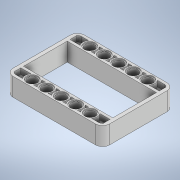
# Autodesk Inventor part: magazine-adapter
Saved by Autodesk Inventor 2021 (Build 250183000, 183)
## iProperties
Created: 2024-03-14
Part Number: magazine-adapter
Material: Generic
Document SubType Name: Modeling
Designer: 22hamfri
Density: 1 g/cm^3
Appearance: Default
Author: 22hamfri
Autodesk Inventor part; units mm, degrees
ref_plane "YZ Plane" through (0, 0, 0) normal (1, 0, 0) x (0, 1, 0)
ref_plane "XZ Plane" through (0, 0, 0) normal (0, 1, 0) x (-1, 0, 0)
ref_plane "XY Plane" through (0, 0, 0) normal (0, 0, 1) x (1, 0, 0)
sketch "Sketch1" plane through (0, 0, 0) normal (0, 1, 0) x (-1, 0, 0)
  line L0 (-24.5, 12) -> (24.5, 12)
  line L1 (24.5, 12) -> (24.5, -12)
  line L2 (24.5, -12) -> (-24.5, -12)
  line L3 (-24.5, -12) -> (-24.5, 12)
  line L4 (-24.5, 12) -> (24.5, -12) construction
  line L5 (24.5, 12) -> (-24.5, -12) construction
  line L6 (-26.5, 19.6) -> (26.5, 19.6)
  line L7 (26.5, 19.6) -> (26.5, -19.6)
  line L8 (26.5, -19.6) -> (-26.5, -19.6)
  line L9 (-26.5, -19.6) -> (-26.5, 19.6)
  line L10 (-26.5, 19.6) -> (26.5, -19.6) construction
  line L11 (26.5, 19.6) -> (-26.5, -19.6) construction
  circle A0 centre (0, -15.8) radius 2.575
  circle A1 centre (0, -15.8) radius 3.1
  circle A2 centre (0, -15.8) radius 3.8
  circle A3 centre (-7.97, -15.8) radius 2.575
  circle A4 centre (-7.97, -15.8) radius 3.1
  circle A5 centre (-7.97, -15.8) radius 3.8
  circle A6 centre (-15.94, -15.8) radius 2.575
  circle A7 centre (-15.94, -15.8) radius 3.1
  circle A8 centre (-15.94, -15.8) radius 3.8
  circle A9 centre (7.97, -15.8) radius 2.575
  circle A10 centre (7.97, -15.8) radius 3.1
  circle A11 centre (7.97, -15.8) radius 3.8
  circle A12 centre (0, -15.8) radius 2.575
  circle A13 centre (0, -15.8) radius 3.1
  circle A14 centre (0, -15.8) radius 3.8
  circle A15 centre (-7.97, -15.8) radius 2.575
  circle A16 centre (-7.97, -15.8) radius 3.1
  circle A17 centre (-7.97, -15.8) radius 3.8
  circle A18 centre (15.94, -15.8) radius 2.575
  circle A19 centre (15.94, -15.8) radius 3.1
  circle A20 centre (15.94, -15.8) radius 3.8
  circle A21 centre (7.97, -15.8) radius 2.575
  circle A22 centre (7.97, -15.8) radius 3.1
  circle A23 centre (7.97, -15.8) radius 3.8
  circle A24 centre (0, -15.8) radius 2.575
  circle A25 centre (0, -15.8) radius 3.1
  circle A26 centre (0, -15.8) radius 3.8
  line L12 (0, 0) -> (0, -19.6)
  line L13 (18.9649, -13.5) -> (24.5, -13.5)
  line L14 (24.5, -13.5) -> (24.5, -17.2318)
  line L15 (12.9151, -13.5) -> (10.9949, -13.5)
  line L16 (12.9151, -18.1) -> (10.9949, -18.1)
  line L17 (4.9451, -13.5) -> (3.0249, -13.5)
  line L18 (4.9451, -18.1) -> (3.0249, -18.1)
  line L19 (-3.0249, -13.5) -> (-4.9451, -13.5)
  line L20 (-3.0249, -18.1) -> (-4.9451, -18.1)
  line L21 (-10.9949, -13.5) -> (-12.9151, -13.5)
  line L22 (-10.9949, -18.1) -> (-12.9151, -18.1)
  line L23 (-18.9649, -13.5) -> (-24.5, -13.5)
  line L24 (-24.5, -13.5) -> (-24.5, -17.2318)
  arc A27 (22.7, -19.6) -> (26.5, -15.8) centre (22.7, -15.8) ccw
  arc A28 (22.7, -18.1) -> (24.5, -17.2318) centre (22.7, -15.8) ccw
  line L25 (22.7, -18.1) -> (18.9649, -18.1)
  arc A29 (-26.5, -15.8) -> (-22.7, -19.6) centre (-22.7, -15.8) ccw
  arc A30 (-24.5, -17.2318) -> (-22.7, -18.1) centre (-22.7, -15.8) ccw
  line L26 (-22.7, -18.1) -> (-18.9649, -18.1)
  line L27 (26.5, 0) -> (-26.5, 0)
  line L28 (24.5, 12) -> (-24.5, 12)
  line L29 (26.5, 19.6) -> (-26.5, 19.6)
  circle A31 centre (0, 15.8) radius 2.575
  circle A32 centre (0, 15.8) radius 3.1
  circle A33 centre (0, 15.8) radius 3.8
  circle A34 centre (-7.97, 15.8) radius 2.575
  circle A35 centre (-7.97, 15.8) radius 3.1
  circle A36 centre (-7.97, 15.8) radius 3.8
  circle A37 centre (-15.94, 15.8) radius 2.575
  circle A38 centre (-15.94, 15.8) radius 3.1
  circle A39 centre (-15.94, 15.8) radius 3.8
  circle A40 centre (7.97, 15.8) radius 2.575
  circle A41 centre (7.97, 15.8) radius 3.1
  circle A42 centre (7.97, 15.8) radius 3.8
  circle A43 centre (0, 15.8) radius 2.575
  circle A44 centre (0, 15.8) radius 3.1
  circle A45 centre (0, 15.8) radius 3.8
  circle A46 centre (-7.97, 15.8) radius 2.575
  circle A47 centre (-7.97, 15.8) radius 3.1
  circle A48 centre (-7.97, 15.8) radius 3.8
  circle A49 centre (15.94, 15.8) radius 2.575
  circle A50 centre (15.94, 15.8) radius 3.1
  circle A51 centre (15.94, 15.8) radius 3.8
  circle A52 centre (7.97, 15.8) radius 2.575
  circle A53 centre (7.97, 15.8) radius 3.1
  circle A54 centre (7.97, 15.8) radius 3.8
  circle A55 centre (0, 15.8) radius 2.575
  circle A56 centre (0, 15.8) radius 3.1
  circle A57 centre (0, 15.8) radius 3.8
  line L30 (18.9649, 13.5) -> (24.5, 13.5)
  line L31 (24.5, 13.5) -> (24.5, 17.2318)
  line L32 (12.9151, 13.5) -> (10.9949, 13.5)
  line L33 (12.9151, 18.1) -> (10.9949, 18.1)
  line L34 (4.9451, 13.5) -> (3.0249, 13.5)
  line L35 (4.9451, 18.1) -> (3.0249, 18.1)
  line L36 (-3.0249, 13.5) -> (-4.9451, 13.5)
  line L37 (-3.0249, 18.1) -> (-4.9451, 18.1)
  line L38 (-10.9949, 13.5) -> (-12.9151, 13.5)
  line L39 (-10.9949, 18.1) -> (-12.9151, 18.1)
  line L40 (-18.9649, 13.5) -> (-24.5, 13.5)
  line L41 (-24.5, 13.5) -> (-24.5, 17.2318)
  arc A58 (26.5, 15.8) -> (22.7, 19.6) centre (22.7, 15.8) ccw
  arc A59 (24.5, 17.2318) -> (22.7, 18.1) centre (22.7, 15.8) ccw
  line L42 (22.7, 18.1) -> (18.9649, 18.1)
  arc A60 (-22.7, 18.1) -> (-24.5, 17.2318) centre (-22.7, 15.8) ccw
  arc A61 (-22.7, 19.6) -> (-26.5, 15.8) centre (-22.7, 15.8) ccw
  line L43 (-22.7, 18.1) -> (-18.9649, 18.1)
  point P0 (0, 0)
  point P1 (0, 19.6)
  dimension "d0" = 24
  dimension "d1" = 49
  dimension "d2" = 2
  dimension "d3" = 5.15
  dimension "d4" = 6.2
  dimension "d5" = 0.7
  dimension "d8" = 7.97
  dimension "d11" = 7.97
  dimension "d14" = 2
  dimension "d15" = 1.5
  dimension "d17" = 3.8
  dimension "d18" = 1.5
  dimension "d19" = 1.5
  constraints: 88 end point, 62 centre point, 56 point on circle, 47 symmetric about line, 12 collinear, 11 parallel, 10 point on line, 9 midpoint, 6 horizontal, 5 perpendicular, 4 tangent, 65 other
  measures "d0" distance between parallel lines of L2 L0
  measures "d1" distance between parallel lines of L1 L3
  measures "d2" distance between parallel lines of L7 L1
  measures "d3" diameter of A0
  measures "d4" diameter of A1
  measures "d5" radial gap between concentric circles of A1 A2
  measures "d8" distance of A0.centre A3.centre
  measures "d11" distance of A0.centre A9.centre
  measures "d14" distance between parallel lines of L3 L9
  measures "d15" distance between parallel lines of L13 L2
  measures "d17" radius of A27
  measures "d18" radial gap between concentric circles of A27 A28
  measures "d19" distance between parallel lines of L8 L25
extrude "Extrusion1" add sketch "Sketch1" against normal mid plane 10 contours L3 L27 L9 A61 L6 A39 L43 A60 L41 L40 L0 | A39 L38 A36 L0 | A39 | L3 L2 A8 L23 L24 A30 L26 L8 A29 L9 L27 | A36 L36 A33 L0 | A36 | A33 L34 A42 L0 | A33 | L2 A5 L21 A8 | A8 | A2 L19 A5 L2 | L2 A11 L17 A2 | L12 A1 A2 | A2 L12 A1 | L27 L7 A27 L8 A20 L25 A28 L14 L13 L2 L1 | L1 L0 A51 L30 L31 A59 L42 L6 A58 L7 L27 | A42 L32 A51 L0 | A42 | L39 A39 L6 A36 | A5 | L2 A20 L15 A11 | A11 | A51 | L37 A36 L6 A33 | A20 | A2 L8 A5 L20 | A8 L22 A5 L8 | L35 A33 L6 A42 | A11 L8 A2 L18 | L33 A42 L6 A51 | A20 L8 A11 L16
extrude "Extrusion2" add sketch "Sketch1" against normal mid plane 9 contours L12 A0 A1 | A1 L12 A0 | A4 | A7 | A10 | A19 | A32 | A35 | A38 | A41 | A50
extrude "Extrusion3" add sketch "Sketch1" along normal mid plane 4 contours L40 L41 A60 L43 A39 | A39 L39 A36 L38 | A36 L37 A33 L36 | A33 L35 A42 L34 | L21 A5 L22 A8 | A8 L26 A30 L24 L23 | L17 A11 L18 A2 | A2 L20 A5 L19 | A42 L33 A51 L32 | L15 A20 L16 A11 | A51 L42 A59 L31 L30 | L13 L14 A28 L25 A20
equation "\"d14\" = d2"
equation "\"d18\" = d15"
equation "\"d19\" = d15"
equation "\"d16\" = d15"
body "Solid1"
